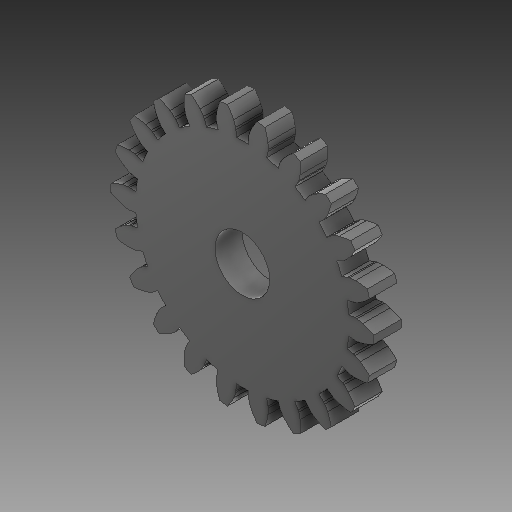
# Autodesk Inventor part: 歯車m2.z22
Saved by Autodesk Inventor 2020 (Build 240168000, 168)
## iProperties
Created: 2019-09-03
Part Number: 歯車m2.z22
Material: アセタール樹脂、黒
Document SubType Name: Modeling
Designer: 雪村
Density: 1.425 g/cm^3
Appearance: 滑らか - 黒
Mass: 6.34973 g
Surface Area: 52.6764 cm^2
Volume: 4.45595 cm^3
Description: ジュラコン 5t
Author: 雪村
Autodesk Inventor part; units mm, degrees
ref_plane "YZ Plane" through (0, 0, 0) normal (1, 0, 0) x (0, 1, 0)
ref_plane "XZ Plane" through (0, 0, 0) normal (0, 1, 0) x (-1, 0, 0)
ref_plane "XY Plane" through (0, 0, 0) normal (0, 0, 1) x (1, 0, 0)
sketch "スケッチ1" plane through (0, 0, 0) normal (0, 0, 1) x (1, 0, 0)
  arc A0 (1.2256, 20.9678) -> (1.1673, 20.6403) centre (3.2398, 20.4403) ccw
  arc A1 (1.5912, 21.9922) -> (1.2256, 20.9678) centre (6.7837, 19.5615) ccw
  arc A2 (2.7153, 23.8459) -> (1.5912, 21.9922) centre (10.6032, 17.7949) ccw
  arc A3 (-4.7313, 20.4638) -> (-4.695, 20.1331) centre (-2.6501, 20.5251) ccw
  arc A4 (-4.6691, 21.5497) -> (-4.7313, 20.4638) centre (0.9978, 20.6803) ccw
  arc A5 (-4.1128, 23.645) -> (-4.6691, 21.5497) centre (5.1603, 20.0614) ccw
  arc A6 (-10.305, 18.3019) -> (-10.1769, 17.9948) centre (-8.3254, 18.9471) ccw
  arc A7 (-10.5512, 19.3613) -> (-10.305, 18.3019) centre (-4.8689, 20.1238) ccw
  arc A8 (-10.6078, 21.5285) -> (-10.5512, 19.3613) centre (-0.7007, 20.7026) ccw
  arc A9 (-15.0438, 14.6573) -> (-14.8344, 14.3987) centre (-13.3261, 15.834) ccw
  arc A10 (-15.5785, 15.6044) -> (-15.0438, 14.6573) centre (-10.3412, 17.9369) ccw
  arc A11 (-16.2434, 17.6679) -> (-15.5785, 15.6044) centre (-6.5049, 19.6666) ccw
  arc A12 (-18.5639, 9.8252) -> (-18.2901, 9.6361) centre (-17.2473, 11.4383) ccw
  arc A13 (-19.3438, 10.5833) -> (-18.5639, 9.8252) centre (-14.9757, 14.2969) ccw
  arc A14 (-20.563, 12.3759) -> (-19.3438, 10.5833) centre (-11.7821, 17.0373) ccw
  arc A15 (-20.58, 4.1972) -> (-20.264, 4.0929) centre (-19.7712, 6.1158) ccw
  arc A16 (-21.5419, 4.7049) -> (-20.58, 4.1972) centre (-18.397, 9.4986) ccw
  arc A17 (-23.2167, 6.0813) -> (-21.5419, 4.7049) centre (-16.1048, 13.0278) ccw
  arc A18 (-20.9288, -1.7709) -> (-20.5963, -1.782) centre (-20.6933, 0.2979) ccw
  arc A19 (-21.9948, -1.5548) -> (-20.9288, -1.7709) centre (-20.3278, 3.9308) ccw
  arc A20 (-23.9896, -0.7059) -> (-21.9948, -1.5548) centre (-19.1228, 7.9628) ccw
  arc A21 (-19.5822, -7.5955) -> (-19.26, -7.5124) centre (-19.939, -5.5442) ccw
  arc A22 (-20.6658, -7.6884) -> (-19.5822, -7.5955) centre (-20.6119, -1.9555) ccw
  arc A23 (-22.819, -7.436) -> (-20.6658, -7.6884) centre (-20.5916, 2.2527) ccw
  arc A24 (-16.649, -12.8047) -> (-16.3633, -12.6343) centre (-17.5694, -10.9371) ccw
  arc A25 (-17.6626, -13.1992) -> (-16.649, -12.8047) centre (-19.226, -7.6833) ccw
  arc A26 (-19.7997, -13.5636) -> (-17.6626, -13.1992) centre (-20.3921, -3.6398) ccw
  arc A27 (-12.3671, -16.9766) -> (-12.141, -16.7326) centre (-13.7764, -15.4439) ccw
  arc A28 (-13.2285, -17.6407) -> (-12.3671, -16.9766) centre (-16.2826, -12.7886) ccw
  arc A29 (-15.1764, -18.5924) -> (-13.2285, -17.6407) centre (-18.5406, -9.2375) ccw
  arc A30 (-7.0833, -19.7732) -> (-6.9351, -19.4753) centre (-8.8673, -18.6996) ccw
  arc A31 (-7.7227, -20.653) -> (-7.0833, -19.7732) centre (-12.0201, -16.858) ccw
  arc A32 (-9.3235, -22.115) -> (-7.7227, -20.653) centre (-15.1871, -14.0868) ccw
  arc A33 (-1.2256, -20.9678) -> (-1.1673, -20.6403) centre (-3.2398, -20.4403) ccw
  arc A34 (-1.5912, -21.9922) -> (-1.2256, -20.9678) centre (-6.7837, -19.5615) ccw
  arc A35 (-2.7153, -23.8459) -> (-1.5912, -21.9922) centre (-10.6032, -17.7949) ccw
  arc A36 (4.7313, -20.4638) -> (4.695, -20.1331) centre (2.6501, -20.5251) ccw
  arc A37 (4.6691, -21.5497) -> (4.7313, -20.4638) centre (-0.9978, -20.6803) ccw
  arc A38 (4.1128, -23.645) -> (4.6691, -21.5497) centre (-5.1603, -20.0614) ccw
  arc A39 (10.305, -18.3019) -> (10.1769, -17.9948) centre (8.3254, -18.9471) ccw
  arc A40 (10.5512, -19.3613) -> (10.305, -18.3019) centre (4.8689, -20.1238) ccw
  arc A41 (10.6078, -21.5285) -> (10.5512, -19.3613) centre (0.7007, -20.7026) ccw
  arc A42 (15.0438, -14.6573) -> (14.8344, -14.3987) centre (13.3261, -15.834) ccw
  arc A43 (15.5785, -15.6044) -> (15.0438, -14.6573) centre (10.3412, -17.9369) ccw
  arc A44 (16.2434, -17.6679) -> (15.5785, -15.6044) centre (6.5049, -19.6666) ccw
  arc A45 (18.5639, -9.8252) -> (18.2901, -9.6361) centre (17.2473, -11.4383) ccw
  arc A46 (19.3438, -10.5833) -> (18.5639, -9.8252) centre (14.9757, -14.2969) ccw
  arc A47 (20.563, -12.3759) -> (19.3438, -10.5833) centre (11.7821, -17.0373) ccw
  arc A48 (20.58, -4.1972) -> (20.264, -4.0929) centre (19.7712, -6.1158) ccw
  arc A49 (21.5419, -4.7049) -> (20.58, -4.1972) centre (18.397, -9.4986) ccw
  arc A50 (23.2167, -6.0813) -> (21.5419, -4.7049) centre (16.1048, -13.0278) ccw
  arc A51 (20.9288, 1.7709) -> (20.5963, 1.782) centre (20.6933, -0.2979) ccw
  arc A52 (21.9948, 1.5548) -> (20.9288, 1.7709) centre (20.3278, -3.9308) ccw
  arc A53 (23.9896, 0.7059) -> (21.9948, 1.5548) centre (19.1228, -7.9628) ccw
  arc A54 (19.5822, 7.5955) -> (19.26, 7.5124) centre (19.939, 5.5442) ccw
  arc A55 (20.6658, 7.6884) -> (19.5822, 7.5955) centre (20.6119, 1.9555) ccw
  arc A56 (22.819, 7.436) -> (20.6658, 7.6884) centre (20.5916, -2.2527) ccw
  arc A57 (16.649, 12.8047) -> (16.3633, 12.6343) centre (17.5694, 10.9371) ccw
  arc A58 (17.6626, 13.1992) -> (16.649, 12.8047) centre (19.226, 7.6833) ccw
  arc A59 (19.7997, 13.5636) -> (17.6626, 13.1992) centre (20.3921, 3.6398) ccw
  arc A60 (12.3671, 16.9766) -> (12.141, 16.7326) centre (13.7764, 15.4439) ccw
  arc A61 (13.2285, 17.6407) -> (12.3671, 16.9766) centre (16.2826, 12.7886) ccw
  arc A62 (15.1764, 18.5924) -> (13.2285, 17.6407) centre (18.5406, 9.2375) ccw
  arc A63 (7.0833, 19.7732) -> (6.9351, 19.4753) centre (8.8673, 18.6996) ccw
  arc A64 (7.7227, 20.653) -> (7.0833, 19.7732) centre (12.0201, 16.858) ccw
  arc A65 (9.3235, 22.115) -> (7.7227, 20.653) centre (15.1871, 14.0868) ccw
  arc A66 (-1.1673, 20.6403) -> (-1.2256, 20.9678) centre (-3.2398, 20.4403) ccw
  arc A67 (-1.2256, 20.9678) -> (-1.5912, 21.9922) centre (-6.7837, 19.5615) ccw
  arc A68 (-1.5912, 21.9922) -> (-2.7153, 23.8459) centre (-10.6032, 17.7949) ccw
  arc A69 (-6.9351, 19.4753) -> (-7.0833, 19.7732) centre (-8.8673, 18.6996) ccw
  arc A70 (-7.0833, 19.7732) -> (-7.7227, 20.653) centre (-12.0201, 16.858) ccw
  arc A71 (-7.7227, 20.653) -> (-9.3235, 22.115) centre (-15.1871, 14.0868) ccw
  arc A72 (-12.141, 16.7326) -> (-12.3671, 16.9766) centre (-13.7764, 15.4439) ccw
  arc A73 (-12.3671, 16.9766) -> (-13.2285, 17.6407) centre (-16.2826, 12.7886) ccw
  arc A74 (-13.2285, 17.6407) -> (-15.1764, 18.5924) centre (-18.5406, 9.2375) ccw
  arc A75 (-16.3633, 12.6343) -> (-16.649, 12.8047) centre (-17.5694, 10.9371) ccw
  arc A76 (-16.649, 12.8047) -> (-17.6626, 13.1992) centre (-19.226, 7.6833) ccw
  arc A77 (-17.6626, 13.1992) -> (-19.7997, 13.5636) centre (-20.3921, 3.6398) ccw
  arc A78 (-19.26, 7.5124) -> (-19.5822, 7.5955) centre (-19.939, 5.5442) ccw
  arc A79 (-19.5822, 7.5955) -> (-20.6658, 7.6884) centre (-20.6119, 1.9555) ccw
  arc A80 (-20.6658, 7.6884) -> (-22.819, 7.436) centre (-20.5916, -2.2527) ccw
  arc A81 (-20.5963, 1.782) -> (-20.9288, 1.7709) centre (-20.6933, -0.2979) ccw
  arc A82 (-20.9288, 1.7709) -> (-21.9948, 1.5548) centre (-20.3278, -3.9308) ccw
  arc A83 (-21.9948, 1.5548) -> (-23.9896, 0.7059) centre (-19.1228, -7.9628) ccw
  arc A84 (-20.264, -4.0929) -> (-20.58, -4.1972) centre (-19.7712, -6.1158) ccw
  arc A85 (-20.58, -4.1972) -> (-21.5419, -4.7049) centre (-18.397, -9.4986) ccw
  arc A86 (-21.5419, -4.7049) -> (-23.2167, -6.0813) centre (-16.1048, -13.0278) ccw
  arc A87 (-18.2901, -9.6361) -> (-18.5639, -9.8252) centre (-17.2473, -11.4383) ccw
  arc A88 (-18.5639, -9.8252) -> (-19.3438, -10.5833) centre (-14.9757, -14.2969) ccw
  arc A89 (-19.3438, -10.5833) -> (-20.563, -12.3759) centre (-11.7821, -17.0373) ccw
  arc A90 (-14.8344, -14.3987) -> (-15.0438, -14.6573) centre (-13.3261, -15.834) ccw
  arc A91 (-15.0438, -14.6573) -> (-15.5785, -15.6044) centre (-10.3412, -17.9369) ccw
  arc A92 (-15.5785, -15.6044) -> (-16.2434, -17.6679) centre (-6.5049, -19.6666) ccw
  arc A93 (-10.1769, -17.9948) -> (-10.305, -18.3019) centre (-8.3254, -18.9471) ccw
  arc A94 (-10.305, -18.3019) -> (-10.5512, -19.3613) centre (-4.8689, -20.1238) ccw
  arc A95 (-10.5512, -19.3613) -> (-10.6078, -21.5285) centre (-0.7007, -20.7026) ccw
  arc A96 (-4.695, -20.1331) -> (-4.7313, -20.4638) centre (-2.6501, -20.5251) ccw
  arc A97 (-4.7313, -20.4638) -> (-4.6691, -21.5497) centre (0.9978, -20.6803) ccw
  arc A98 (-4.6691, -21.5497) -> (-4.1128, -23.645) centre (5.1603, -20.0614) ccw
  arc A99 (1.1673, -20.6403) -> (1.2256, -20.9678) centre (3.2398, -20.4403) ccw
  arc A100 (1.2256, -20.9678) -> (1.5912, -21.9922) centre (6.7837, -19.5615) ccw
  arc A101 (1.5912, -21.9922) -> (2.7153, -23.8459) centre (10.6032, -17.7949) ccw
  arc A102 (6.9351, -19.4753) -> (7.0833, -19.7732) centre (8.8673, -18.6996) ccw
  arc A103 (7.0833, -19.7732) -> (7.7227, -20.653) centre (12.0201, -16.858) ccw
  arc A104 (7.7227, -20.653) -> (9.3235, -22.115) centre (15.1871, -14.0868) ccw
  arc A105 (12.141, -16.7326) -> (12.3671, -16.9766) centre (13.7764, -15.4439) ccw
  arc A106 (12.3671, -16.9766) -> (13.2285, -17.6407) centre (16.2826, -12.7886) ccw
  arc A107 (13.2285, -17.6407) -> (15.1764, -18.5924) centre (18.5406, -9.2375) ccw
  arc A108 (16.3633, -12.6343) -> (16.649, -12.8047) centre (17.5694, -10.9371) ccw
  arc A109 (16.649, -12.8047) -> (17.6626, -13.1992) centre (19.226, -7.6833) ccw
  arc A110 (17.6626, -13.1992) -> (19.7997, -13.5636) centre (20.3921, -3.6398) ccw
  arc A111 (19.26, -7.5124) -> (19.5822, -7.5955) centre (19.939, -5.5442) ccw
  arc A112 (19.5822, -7.5955) -> (20.6658, -7.6884) centre (20.6119, -1.9555) ccw
  arc A113 (20.6658, -7.6884) -> (22.819, -7.436) centre (20.5916, 2.2527) ccw
  arc A114 (20.5963, -1.782) -> (20.9288, -1.7709) centre (20.6933, 0.2979) ccw
  arc A115 (20.9288, -1.7709) -> (21.9948, -1.5548) centre (20.3278, 3.9308) ccw
  arc A116 (21.9948, -1.5548) -> (23.9896, -0.7059) centre (19.1228, 7.9628) ccw
  arc A117 (20.264, 4.0929) -> (20.58, 4.1972) centre (19.7712, 6.1158) ccw
  arc A118 (20.58, 4.1972) -> (21.5419, 4.7049) centre (18.397, 9.4986) ccw
  arc A119 (21.5419, 4.7049) -> (23.2167, 6.0813) centre (16.1048, 13.0278) ccw
  arc A120 (18.2901, 9.6361) -> (18.5639, 9.8252) centre (17.2473, 11.4383) ccw
  arc A121 (18.5639, 9.8252) -> (19.3438, 10.5833) centre (14.9757, 14.2969) ccw
  arc A122 (19.3438, 10.5833) -> (20.563, 12.3759) centre (11.7821, 17.0373) ccw
  arc A123 (14.8344, 14.3987) -> (15.0438, 14.6573) centre (13.3261, 15.834) ccw
  arc A124 (15.0438, 14.6573) -> (15.5785, 15.6044) centre (10.3412, 17.9369) ccw
  arc A125 (15.5785, 15.6044) -> (16.2434, 17.6679) centre (6.5049, 19.6666) ccw
  arc A126 (10.1769, 17.9948) -> (10.305, 18.3019) centre (8.3254, 18.9471) ccw
  arc A127 (10.305, 18.3019) -> (10.5512, 19.3613) centre (4.8689, 20.1238) ccw
  arc A128 (10.5512, 19.3613) -> (10.6078, 21.5285) centre (0.7007, 20.7026) ccw
  arc A129 (4.695, 20.1331) -> (4.7313, 20.4638) centre (2.6501, 20.5251) ccw
  arc A130 (4.7313, 20.4638) -> (4.6691, 21.5497) centre (-0.9978, 20.6803) ccw
  arc A131 (4.6691, 21.5497) -> (4.1128, 23.645) centre (-5.1603, 20.0614) ccw
  arc A132 (1.1011, 19.4689) -> (-1.1011, 19.4689) centre (0, 0) ccw
  arc A133 (-4.4285, 18.9905) -> (-6.5415, 18.3701) centre (0, 0) ccw
  arc A134 (-9.5994, 16.9736) -> (-11.452, 15.783) centre (0, 0) ccw
  arc A135 (-13.9926, 13.5815) -> (-15.4347, 11.9173) centre (0, 0) ccw
  arc A136 (-17.2521, 9.0892) -> (-18.1669, 7.0861) centre (0, 0) ccw
  arc A137 (-19.114, 3.8606) -> (-19.4274, 1.6808) centre (0, 0) ccw
  arc A138 (-19.4274, -1.6808) -> (-19.114, -3.8606) centre (0, 0) ccw
  arc A139 (-18.1669, -7.0861) -> (-17.2521, -9.0892) centre (0, 0) ccw
  arc A140 (-15.4347, -11.9173) -> (-13.9926, -13.5815) centre (0, 0) ccw
  arc A141 (-11.452, -15.783) -> (-9.5994, -16.9736) centre (0, 0) ccw
  arc A142 (-6.5415, -18.3701) -> (-4.4285, -18.9905) centre (0, 0) ccw
  arc A143 (-1.1011, -19.4689) -> (1.1011, -19.4689) centre (0, 0) ccw
  arc A144 (4.4285, -18.9905) -> (6.5415, -18.3701) centre (0, 0) ccw
  arc A145 (9.5994, -16.9736) -> (11.452, -15.783) centre (0, 0) ccw
  arc A146 (13.9926, -13.5815) -> (15.4347, -11.9173) centre (0, 0) ccw
  arc A147 (17.2521, -9.0892) -> (18.1669, -7.0861) centre (0, 0) ccw
  arc A148 (19.114, -3.8606) -> (19.4274, -1.6808) centre (0, 0) ccw
  arc A149 (19.4274, 1.6808) -> (19.114, 3.8606) centre (0, 0) ccw
  arc A150 (18.1669, 7.0861) -> (17.2521, 9.0892) centre (0, 0) ccw
  arc A151 (15.4347, 11.9173) -> (13.9926, 13.5815) centre (0, 0) ccw
  arc A152 (11.452, 15.783) -> (9.5994, 16.9736) centre (0, 0) ccw
  arc A153 (6.5415, 18.3701) -> (4.4285, 18.9905) centre (0, 0) ccw
  arc A154 (-2.7153, 23.8459) -> (-4.1128, 23.645) centre (0, 0) ccw
  arc A155 (-9.3235, 22.115) -> (-10.6078, 21.5285) centre (0, 0) ccw
  arc A156 (-15.1764, 18.5924) -> (-16.2434, 17.6679) centre (0, 0) ccw
  arc A157 (-19.7997, 13.5636) -> (-20.563, 12.3759) centre (0, 0) ccw
  arc A158 (-22.819, 7.436) -> (-23.2167, 6.0813) centre (0, 0) ccw
  arc A159 (-23.9896, 0.7059) -> (-23.9896, -0.7059) centre (0, 0) ccw
  arc A160 (-23.2167, -6.0813) -> (-22.819, -7.436) centre (0, 0) ccw
  arc A161 (-20.563, -12.3759) -> (-19.7997, -13.5636) centre (0, 0) ccw
  arc A162 (-16.2434, -17.6679) -> (-15.1764, -18.5924) centre (0, 0) ccw
  arc A163 (-10.6078, -21.5285) -> (-9.3235, -22.115) centre (0, 0) ccw
  arc A164 (-4.1128, -23.645) -> (-2.7153, -23.8459) centre (0, 0) ccw
  arc A165 (2.7153, -23.8459) -> (4.1128, -23.645) centre (0, 0) ccw
  arc A166 (9.3235, -22.115) -> (10.6078, -21.5285) centre (0, 0) ccw
  arc A167 (15.1764, -18.5924) -> (16.2434, -17.6679) centre (0, 0) ccw
  arc A168 (19.7997, -13.5636) -> (20.563, -12.3759) centre (0, 0) ccw
  arc A169 (22.819, -7.436) -> (23.2167, -6.0813) centre (0, 0) ccw
  arc A170 (23.9896, -0.7059) -> (23.9896, 0.7059) centre (0, 0) ccw
  arc A171 (23.2167, 6.0813) -> (22.819, 7.436) centre (0, 0) ccw
  arc A172 (20.563, 12.3759) -> (19.7997, 13.5636) centre (0, 0) ccw
  arc A173 (16.2434, 17.6679) -> (15.1764, 18.5924) centre (0, 0) ccw
  arc A174 (10.6078, 21.5285) -> (9.3235, 22.115) centre (0, 0) ccw
  arc A175 (4.1128, 23.645) -> (2.7153, 23.8459) centre (0, 0) ccw
  line L0 (1.1011, 19.4689) -> (1.1673, 20.6403)
  line L1 (-4.4285, 18.9905) -> (-4.695, 20.1331)
  line L2 (-9.5994, 16.9736) -> (-10.1769, 17.9948)
  line L3 (-13.9926, 13.5815) -> (-14.8344, 14.3987)
  line L4 (-17.2521, 9.0892) -> (-18.2901, 9.6361)
  line L5 (-19.114, 3.8606) -> (-20.264, 4.0929)
  line L6 (-19.4274, -1.6808) -> (-20.5963, -1.782)
  line L7 (-18.1669, -7.0861) -> (-19.26, -7.5124)
  line L8 (-15.4347, -11.9173) -> (-16.3633, -12.6343)
  line L9 (-11.452, -15.783) -> (-12.141, -16.7326)
  line L10 (-6.5415, -18.3701) -> (-6.9351, -19.4753)
  line L11 (-1.1011, -19.4689) -> (-1.1673, -20.6403)
  line L12 (4.4285, -18.9905) -> (4.695, -20.1331)
  line L13 (9.5994, -16.9736) -> (10.1769, -17.9948)
  line L14 (13.9926, -13.5815) -> (14.8344, -14.3987)
  line L15 (17.2521, -9.0892) -> (18.2901, -9.6361)
  line L16 (19.114, -3.8606) -> (20.264, -4.0929)
  line L17 (19.4274, 1.6808) -> (20.5963, 1.782)
  line L18 (18.1669, 7.0861) -> (19.26, 7.5124)
  line L19 (15.4347, 11.9173) -> (16.3633, 12.6343)
  line L20 (11.452, 15.783) -> (12.141, 16.7326)
  line L21 (6.5415, 18.3701) -> (6.9351, 19.4753)
  line L22 (-1.1011, 19.4689) -> (-1.1673, 20.6403)
  line L23 (-6.5415, 18.3701) -> (-6.9351, 19.4753)
  line L24 (-11.452, 15.783) -> (-12.141, 16.7326)
  line L25 (-15.4347, 11.9173) -> (-16.3633, 12.6343)
  line L26 (-18.1669, 7.0861) -> (-19.26, 7.5124)
  line L27 (-19.4274, 1.6808) -> (-20.5963, 1.782)
  line L28 (-19.114, -3.8606) -> (-20.264, -4.0929)
  line L29 (-17.2521, -9.0892) -> (-18.2901, -9.6361)
  line L30 (-13.9926, -13.5815) -> (-14.8344, -14.3987)
  line L31 (-9.5994, -16.9736) -> (-10.1769, -17.9948)
  line L32 (-4.4285, -18.9905) -> (-4.695, -20.1331)
  line L33 (1.1011, -19.4689) -> (1.1673, -20.6403)
  line L34 (6.5415, -18.3701) -> (6.9351, -19.4753)
  line L35 (11.452, -15.783) -> (12.141, -16.7326)
  line L36 (15.4347, -11.9173) -> (16.3633, -12.6343)
  line L37 (18.1669, -7.0861) -> (19.26, -7.5124)
  line L38 (19.4274, -1.6808) -> (20.5963, -1.782)
  line L39 (19.114, 3.8606) -> (20.264, 4.0929)
  line L40 (17.2521, 9.0892) -> (18.2901, 9.6361)
  line L41 (13.9926, 13.5815) -> (14.8344, 14.3987)
  line L42 (9.5994, 16.9736) -> (10.1769, 17.9948)
  line L43 (4.4285, 18.9905) -> (4.695, 20.1331)
  line L44 (-26, 0) -> (26, 0)
  line L45 (0, -26) -> (0, 26)
  line L46 (44, 24) -> (114, 24)
  line L47 (44, 16) -> (114, 16)
  line L48 (44, 8) -> (114, 8)
  line L49 (44, 0) -> (114, 0)
  line L50 (44, -8) -> (114, -8)
  line L51 (44, -16) -> (114, -16)
  line L52 (44, -24) -> (114, -24)
  line L53 (44, -32) -> (114, -32)
  line L54 (44, -40) -> (114, -40)
  line L55 (44, -48) -> (114, -48)
  line L56 (44, -56) -> (114, -56)
  line L57 (44, -64) -> (114, -64)
  line L58 (44, -72) -> (114, -72)
  line L59 (44, 24) -> (44, -72)
  line L60 (114, 24) -> (114, -72)
  line L61 (79, 16) -> (79, -72)
  point P0 (0, 0)
  point P1 (50, 18)
  point P2 (52.5, 10)
  point P3 (52.5, 2)
  point P4 (50, -6)
  point P5 (52.5, -14)
  point P6 (47.5, -22)
  point P7 (50, -30)
  point P8 (50, -38)
  point P9 (50, -46)
  point P10 (52.5, -54)
  point P11 (52.5, -62)
  point P12 (50, -70)
  point P13 (80, 10)
  point P14 (95, 2)
  point P15 (96.25, -6)
  point P16 (92.5, -14)
  point P17 (95, -22)
  point P18 (88.75, -30)
  point P19 (95, -38)
  point P20 (95, -46)
  point P21 (90, -54)
  point P22 (1, 39.5)
  point P23 (1, 33.5)
  point P24 (17.1875, 39.5)
  point P25 (19.3125, 33.5)
  constraints: 264 point on circle, 132 centre point, 120 end point, 14 horizontal, 2 horizontal alignment, 2 midpoint, 2 vertical, 2 vertical alignment, 767 other
extrude "押し出し1" add sketch "スケッチ1" along normal blind 5 contours A1 A2 A175 A131 A130 A129 L43 A153 L21 A63 A64 A65 A174 A128 A127 A126 L42 A152 L20 A60 A61 A62 A173 A125 A124 A123 L41 A151 L19 A57 A58 A59 A172 A122 A121 A120 L40 A150 L18 A54 A55 A56 A171 A119 A118 A117 L39 A149 L17 A51 A52 A53 A170 L44 L45 A132 L0 A0 | L45 L44 A159 A83 A82 A81 L27 A137 L5 A15 A16 A17 A158 A80 A79 A78 L26 A136 L4 A12 A13 A14 A157 A77 A76 A75 L25 A135 L3 A9 A10 A11 A156 A74 A73 A72 L24 A134 L2 A6 A7 A8 A155 A71 A70 A69 L23 A133 L1 A3 A4 A5 A154 A68 A67 A66 L22 A132 | L45 A143 L11 A33 A34 A35 A164 A98 A97 A96 L32 A142 L10 A30 A31 A32 A163 A95 A94 A93 L31 A141 L9 A27 A28 A29 A162 A92 A91 A90 L30 A140 L8 A24 A25 A26 A161 A89 A88 A87 L29 A139 L7 A21 A22 A23 A160 A86 A85 A84 L28 A138 L6 A18 A19 A20 A159 L44 | L44 A170 A116 A115 A114 L38 A148 L16 A48 A49 A50 A169 A113 A112 A111 L37 A147 L15 A45 A46 A47 A168 A110 A109 A108 L36 A146 L14 A42 A43 A44 A167 A107 A106 A105 L35 A145 L13 A39 A40 A41 A166 A104 A103 A102 L34 A144 L12 A36 A37 A38 A165 A101 A100 A99 L33 A143 L45
sketch "スケッチ2" plane through (0, 0, 5) normal (0, 0, 1) x (1, 0, 0)
  circle A0 centre (0, 0) radius 5
  dimension "d2" = 10
  constraints: 1 centre point, 1 coincident
  measures "d2" diameter of A0
extrude "押し出し2" cut sketch "スケッチ2" against normal through all
sketch "スケッチ3" plane through (0, 0, 5) normal (0, 0, 1) x (1, 0, 0)
  circle A0 centre (0, 0) radius 8
  circle A1 centre (0, 0) radius 5
  circle A2 centre (0, 0) radius 17
  line L0 (0, 15.6403) -> (0, -15.6403)
  line L1 (-15.4429, 0) -> (15.4429, 0)
  line L2 (-1, 16.9706) -> (-1.5, 7.8581)
  line L3 (1, 16.9706) -> (1.5, 7.8581)
  line L4 (7.8581, 1.5) -> (16.9706, 1)
  line L5 (7.8581, -1.5) -> (16.9706, -1)
  circle A3 centre (0, 0) radius 8
  line L6 (1.5, -7.8581) -> (1, -16.9706)
  line L7 (-16.9706, 1) -> (-7.8581, 1.5)
  line L8 (-16.9706, -1) -> (-7.8581, -1.5)
  line L9 (-1.5, -7.8581) -> (-1, -16.9706)
  circle A4 centre (0, 0) radius 5 projected
  circle A5 centre (0, 0) radius 19.5
  point P0 (16.9761, 62.7038)
  point P1 (20.9761, 62.7038)
  point P2 (11.2302, 68.4498)
  point P3 (11.2302, 72.4498)
  point P4 (16.9761, 62.7038)
  point P5 (20.9761, 62.7038)
  point P6 (11.2302, 68.4498)
  point P7 (11.2302, 72.4498)
  point P8 (-6.5415, 18.3701)
  point P9 (-1.5, -7.8581)
  point P10 (1.5, -7.8581)
  point P11 (-7.8581, -1.5)
  point P12 (-7.8581, 1.5)
  dimension "d40" = 2.5
  dimension "d24" = 1
  dimension "d25" = 1
  dimension "d26" = 1
  dimension "d27" = 1
  dimension "d28" = 1
  dimension "d29" = 1
  dimension "d30" = 1
  dimension "d31" = 1
  dimension "d32" = 1.5
  dimension "d33" = 1.5
  dimension "d34" = 1.5
  dimension "d35" = 1.5
  dimension "d36" = 1.5
  dimension "d37" = 1.5
  dimension "d38" = 1.5
  dimension "d39" = 1.5
  dimension "d41" = 3
  constraints: 20 end point, 4 point on circle, 3 concentric, 2 centre point, 2 coincident, 2 midpoint, 1 horizontal, 1 vertical, 22 other
  measures "d24" distance from line of L0 L2.start
  measures "d25" distance from line of L3.start L0
  measures "d26" distance from line of L1 L4.end
  measures "d27" distance from line of L5.end L1
  measures "d28" distance from line of L0 L6.end
  measures "d29" distance from line of L0 L9.end
  measures "d30" distance from line of L1 L8.start
  measures "d31" distance from line of L1 L7.start
  measures "d32" distance from line of L0 L2.end
  measures "d33" distance from line of L0 L3.end
  measures "d34" distance from line of L1 L4.start
  measures "d35" distance from line of L5.start L1
  measures "d36" distance from line of L0 L6.start
  measures "d37" distance from line of L9.start L0
  measures "d38" distance from line of L1 L8.end
  measures "d39" distance from line of L1 L7.end
  measures "d41" radial gap between concentric circles of A0 A1
extrude "押し出し3" cut sketch "スケッチ3" against normal through all contours A0 L3 A2 L4 | L5 A2 L6 A0 | A0 L7 A2 L2 | L9 A2 L8 A0
fillet "フィレット1" radius 2 16 edges at (-16.9706, 1, 2.5) (-16.9706, -1, 2.5) (-7.8581, -1.5, 2.5) (-7.8581, 1.5, 2.5) (-1.5, 7.8581, 2.5) (1.5, 7.8581, 2.5) (16.9706, 1, 2.5) (16.9706, -1, 2.5) (7.8581, -1.5, 2.5) (7.8581, 1.5, 2.5) (1.5, -7.8581, 2.5) (-1.5, -7.8581, 2.5) (-1, -16.9706, 2.5) (1, -16.9706, 2.5) (-1, 16.9706, 2.5) (1, 16.9706, 2.5)
sketch "スケッチ4" plane through (0, 0, 5) normal (0, 0, 1) x (1, 0, 0)
  line L0 (9.288, -1.4215) -> (14.5604, -1.1322) projected
  arc A0 (16.626, -3.5465) -> (14.5604, -1.1322) centre (14.67, -3.1292) ccw projected
  arc A1 (3.5465, -16.626) -> (16.626, -3.5465) centre (0, 0) ccw projected
  arc A2 (1.1322, -14.5604) -> (3.5465, -16.626) centre (3.1292, -14.67) ccw projected
  line L1 (1.1322, -14.5604) -> (1.4215, -9.288) projected
  arc A3 (2.7348, -7.518) -> (1.4215, -9.288) centre (3.4185, -9.3975) ccw projected
  arc A4 (2.7348, -7.518) -> (7.518, -2.7348) centre (0, 0) ccw projected
  arc A5 (9.288, -1.4215) -> (7.518, -2.7348) centre (9.3975, -3.4185) ccw projected
  arc A6 (16.626, 3.5465) -> (3.5465, 16.626) centre (0, 0) ccw projected
  arc A7 (14.5604, 1.1322) -> (16.626, 3.5465) centre (14.67, 3.1292) ccw projected
  line L2 (14.5604, 1.1322) -> (9.288, 1.4215) projected
  arc A8 (7.518, 2.7348) -> (9.288, 1.4215) centre (9.3975, 3.4185) ccw projected
  arc A9 (7.518, 2.7348) -> (2.7348, 7.518) centre (0, 0) ccw projected
  arc A10 (1.4215, 9.288) -> (2.7348, 7.518) centre (3.4185, 9.3975) ccw projected
  line L3 (1.4215, 9.288) -> (1.1322, 14.5604) projected
  arc A11 (3.5465, 16.626) -> (1.1322, 14.5604) centre (3.1292, 14.67) ccw projected
  arc A12 (-7.518, -2.7348) -> (-2.7348, -7.518) centre (0, 0) ccw projected
  arc A13 (-1.4215, -9.288) -> (-2.7348, -7.518) centre (-3.4185, -9.3975) ccw projected
  line L4 (-1.4215, -9.288) -> (-1.1322, -14.5604) projected
  arc A14 (-3.5465, -16.626) -> (-1.1322, -14.5604) centre (-3.1292, -14.67) ccw projected
  arc A15 (-16.626, -3.5465) -> (-3.5465, -16.626) centre (0, 0) ccw projected
  arc A16 (-14.5604, -1.1322) -> (-16.626, -3.5465) centre (-14.67, -3.1292) ccw projected
  line L5 (-14.5604, -1.1322) -> (-9.288, -1.4215) projected
  arc A17 (-7.518, -2.7348) -> (-9.288, -1.4215) centre (-9.3975, -3.4185) ccw projected
  line L6 (-1.1322, 14.5604) -> (-1.4215, 9.288) projected
  arc A18 (-2.7348, 7.518) -> (-1.4215, 9.288) centre (-3.4185, 9.3975) ccw projected
  arc A19 (-2.7348, 7.518) -> (-7.518, 2.7348) centre (0, 0) ccw projected
  arc A20 (-9.288, 1.4215) -> (-7.518, 2.7348) centre (-9.3975, 3.4185) ccw projected
  line L7 (-9.288, 1.4215) -> (-14.5604, 1.1322) projected
  arc A21 (-16.626, 3.5465) -> (-14.5604, 1.1322) centre (-14.67, 3.1292) ccw projected
  arc A22 (-3.5465, 16.626) -> (-16.626, 3.5465) centre (0, 0) ccw projected
  arc A23 (-1.1322, 14.5604) -> (-3.5465, 16.626) centre (-3.1292, 14.67) ccw projected
  circle A24 centre (0, 0) radius 5 projected
  arc A25 (-9.3235, 22.115) -> (-10.6078, 21.5285) centre (0, 0) ccw projected
  arc A26 (-10.6078, 21.5285) -> (-10.5512, 19.3613) centre (-0.7007, 20.7026) ccw projected
  arc A27 (-10.5512, 19.3613) -> (-10.305, 18.3019) centre (-4.8689, 20.1238) ccw projected
  arc A28 (-10.305, 18.3019) -> (-10.1769, 17.9948) centre (-8.3254, 18.9471) ccw projected
  line L8 (-10.1769, 17.9948) -> (-9.5994, 16.9736) projected
  arc A29 (-9.5994, 16.9736) -> (-11.452, 15.783) centre (0, 0) ccw projected
  line L9 (-11.452, 15.783) -> (-12.141, 16.7326) projected
  arc A30 (-12.141, 16.7326) -> (-12.3671, 16.9766) centre (-13.7764, 15.4439) ccw projected
  arc A31 (-12.3671, 16.9766) -> (-13.2285, 17.6407) centre (-16.2826, 12.7886) ccw projected
  arc A32 (-13.2285, 17.6407) -> (-15.1764, 18.5924) centre (-18.5406, 9.2375) ccw projected
  arc A33 (-15.1764, 18.5924) -> (-16.2434, 17.6679) centre (0, 0) ccw projected
  arc A34 (-16.2434, 17.6679) -> (-15.5785, 15.6044) centre (-6.5049, 19.6666) ccw projected
  arc A35 (-15.5785, 15.6044) -> (-15.0438, 14.6573) centre (-10.3412, 17.9369) ccw projected
  arc A36 (-15.0438, 14.6573) -> (-14.8344, 14.3987) centre (-13.3261, 15.834) ccw projected
  line L10 (-14.8344, 14.3987) -> (-13.9926, 13.5815) projected
  arc A37 (-13.9926, 13.5815) -> (-15.4347, 11.9173) centre (0, 0) ccw projected
  line L11 (-15.4347, 11.9173) -> (-16.3633, 12.6343) projected
  arc A38 (-16.3633, 12.6343) -> (-16.649, 12.8047) centre (-17.5694, 10.9371) ccw projected
  arc A39 (-16.649, 12.8047) -> (-17.6626, 13.1992) centre (-19.226, 7.6833) ccw projected
  arc A40 (-17.6626, 13.1992) -> (-19.7997, 13.5636) centre (-20.3921, 3.6398) ccw projected
  arc A41 (-19.7997, 13.5636) -> (-20.563, 12.3759) centre (0, 0) ccw projected
  arc A42 (-20.563, 12.3759) -> (-19.3438, 10.5833) centre (-11.7821, 17.0373) ccw projected
  arc A43 (-19.3438, 10.5833) -> (-18.5639, 9.8252) centre (-14.9757, 14.2969) ccw projected
  arc A44 (-18.5639, 9.8252) -> (-18.2901, 9.6361) centre (-17.2473, 11.4383) ccw projected
  line L12 (-18.2901, 9.6361) -> (-17.2521, 9.0892) projected
  arc A45 (-17.2521, 9.0892) -> (-18.1669, 7.0861) centre (0, 0) ccw projected
  line L13 (-18.1669, 7.0861) -> (-19.26, 7.5124) projected
  arc A46 (-19.26, 7.5124) -> (-19.5822, 7.5955) centre (-19.939, 5.5442) ccw projected
  arc A47 (-19.5822, 7.5955) -> (-20.6658, 7.6884) centre (-20.6119, 1.9555) ccw projected
  arc A48 (-20.6658, 7.6884) -> (-22.819, 7.436) centre (-20.5916, -2.2527) ccw projected
  arc A49 (-22.819, 7.436) -> (-23.2167, 6.0813) centre (0, 0) ccw projected
  arc A50 (-23.2167, 6.0813) -> (-21.5419, 4.7049) centre (-16.1048, 13.0278) ccw projected
  arc A51 (-21.5419, 4.7049) -> (-20.58, 4.1972) centre (-18.397, 9.4986) ccw projected
  arc A52 (-20.58, 4.1972) -> (-20.264, 4.0929) centre (-19.7712, 6.1158) ccw projected
  line L14 (-20.264, 4.0929) -> (-19.114, 3.8606) projected
  arc A53 (-19.114, 3.8606) -> (-19.4274, 1.6808) centre (0, 0) ccw projected
  line L15 (-19.4274, 1.6808) -> (-20.5963, 1.782) projected
  arc A54 (-20.5963, 1.782) -> (-20.9288, 1.7709) centre (-20.6933, -0.2979) ccw projected
  arc A55 (-20.9288, 1.7709) -> (-21.9948, 1.5548) centre (-20.3278, -3.9308) ccw projected
  arc A56 (-21.9948, 1.5548) -> (-23.9896, 0.7059) centre (-19.1228, -7.9628) ccw projected
  arc A57 (-23.9896, 0.7059) -> (-23.9896, -0.7059) centre (0, 0) ccw projected
  arc A58 (-23.9896, -0.7059) -> (-21.9948, -1.5548) centre (-19.1228, 7.9628) ccw projected
  arc A59 (-21.9948, -1.5548) -> (-20.9288, -1.7709) centre (-20.3278, 3.9308) ccw projected
  arc A60 (-20.9288, -1.7709) -> (-20.5963, -1.782) centre (-20.6933, 0.2979) ccw projected
  line L16 (-20.5963, -1.782) -> (-19.4274, -1.6808) projected
  arc A61 (-19.4274, -1.6808) -> (-19.114, -3.8606) centre (0, 0) ccw projected
  line L17 (-19.114, -3.8606) -> (-20.264, -4.0929) projected
  arc A62 (-20.264, -4.0929) -> (-20.58, -4.1972) centre (-19.7712, -6.1158) ccw projected
  arc A63 (-20.58, -4.1972) -> (-21.5419, -4.7049) centre (-18.397, -9.4986) ccw projected
  arc A64 (-21.5419, -4.7049) -> (-23.2167, -6.0813) centre (-16.1048, -13.0278) ccw projected
  arc A65 (-23.2167, -6.0813) -> (-22.819, -7.436) centre (0, 0) ccw projected
  arc A66 (-22.819, -7.436) -> (-20.6658, -7.6884) centre (-20.5916, 2.2527) ccw projected
  arc A67 (-20.6658, -7.6884) -> (-19.5822, -7.5955) centre (-20.6119, -1.9555) ccw projected
  arc A68 (-19.5822, -7.5955) -> (-19.26, -7.5124) centre (-19.939, -5.5442) ccw projected
  line L18 (-19.26, -7.5124) -> (-18.1669, -7.0861) projected
  arc A69 (-18.1669, -7.0861) -> (-17.2521, -9.0892) centre (0, 0) ccw projected
  line L19 (-17.2521, -9.0892) -> (-18.2901, -9.6361) projected
  arc A70 (-18.2901, -9.6361) -> (-18.5639, -9.8252) centre (-17.2473, -11.4383) ccw projected
  arc A71 (-18.5639, -9.8252) -> (-19.3438, -10.5833) centre (-14.9757, -14.2969) ccw projected
  arc A72 (-19.3438, -10.5833) -> (-20.563, -12.3759) centre (-11.7821, -17.0373) ccw projected
  arc A73 (-20.563, -12.3759) -> (-19.7997, -13.5636) centre (0, 0) ccw projected
  arc A74 (-19.7997, -13.5636) -> (-17.6626, -13.1992) centre (-20.3921, -3.6398) ccw projected
  arc A75 (-17.6626, -13.1992) -> (-16.649, -12.8047) centre (-19.226, -7.6833) ccw projected
  arc A76 (-16.649, -12.8047) -> (-16.3633, -12.6343) centre (-17.5694, -10.9371) ccw projected
  line L20 (-16.3633, -12.6343) -> (-15.4347, -11.9173) projected
  arc A77 (-15.4347, -11.9173) -> (-13.9926, -13.5815) centre (0, 0) ccw projected
  line L21 (-13.9926, -13.5815) -> (-14.8344, -14.3987) projected
  arc A78 (-14.8344, -14.3987) -> (-15.0438, -14.6573) centre (-13.3261, -15.834) ccw projected
  arc A79 (-15.0438, -14.6573) -> (-15.5785, -15.6044) centre (-10.3412, -17.9369) ccw projected
  arc A80 (-15.5785, -15.6044) -> (-16.2434, -17.6679) centre (-6.5049, -19.6666) ccw projected
  arc A81 (-16.2434, -17.6679) -> (-15.1764, -18.5924) centre (0, 0) ccw projected
  arc A82 (-15.1764, -18.5924) -> (-13.2285, -17.6407) centre (-18.5406, -9.2375) ccw projected
  arc A83 (-13.2285, -17.6407) -> (-12.3671, -16.9766) centre (-16.2826, -12.7886) ccw projected
  arc A84 (-12.3671, -16.9766) -> (-12.141, -16.7326) centre (-13.7764, -15.4439) ccw projected
  line L22 (-12.141, -16.7326) -> (-11.452, -15.783) projected
  arc A85 (-11.452, -15.783) -> (-9.5994, -16.9736) centre (0, 0) ccw projected
  line L23 (-9.5994, -16.9736) -> (-10.1769, -17.9948) projected
  arc A86 (-10.1769, -17.9948) -> (-10.305, -18.3019) centre (-8.3254, -18.9471) ccw projected
  arc A87 (-10.305, -18.3019) -> (-10.5512, -19.3613) centre (-4.8689, -20.1238) ccw projected
  arc A88 (-10.5512, -19.3613) -> (-10.6078, -21.5285) centre (-0.7007, -20.7026) ccw projected
  arc A89 (-10.6078, -21.5285) -> (-9.3235, -22.115) centre (0, 0) ccw projected
  arc A90 (-9.3235, -22.115) -> (-7.7227, -20.653) centre (-15.1871, -14.0868) ccw projected
  arc A91 (-7.7227, -20.653) -> (-7.0833, -19.7732) centre (-12.0201, -16.858) ccw projected
  arc A92 (-7.0833, -19.7732) -> (-6.9351, -19.4753) centre (-8.8673, -18.6996) ccw projected
  line L24 (-6.9351, -19.4753) -> (-6.5415, -18.3701) projected
  arc A93 (-6.5415, -18.3701) -> (-4.4285, -18.9905) centre (0, 0) ccw projected
  line L25 (-4.4285, -18.9905) -> (-4.695, -20.1331) projected
  arc A94 (-4.695, -20.1331) -> (-4.7313, -20.4638) centre (-2.6501, -20.5251) ccw projected
  arc A95 (-4.7313, -20.4638) -> (-4.6691, -21.5497) centre (0.9978, -20.6803) ccw projected
  arc A96 (-4.6691, -21.5497) -> (-4.1128, -23.645) centre (5.1603, -20.0614) ccw projected
  arc A97 (-4.1128, -23.645) -> (-2.7153, -23.8459) centre (0, 0) ccw projected
  arc A98 (-2.7153, -23.8459) -> (-1.5912, -21.9922) centre (-10.6032, -17.7949) ccw projected
  arc A99 (-1.5912, -21.9922) -> (-1.2256, -20.9678) centre (-6.7837, -19.5615) ccw projected
  arc A100 (-1.2256, -20.9678) -> (-1.1673, -20.6403) centre (-3.2398, -20.4403) ccw projected
  line L26 (-1.1673, -20.6403) -> (-1.1011, -19.4689) projected
  arc A101 (-1.1011, -19.4689) -> (1.1011, -19.4689) centre (0, 0) ccw projected
  line L27 (1.1011, -19.4689) -> (1.1673, -20.6403) projected
  arc A102 (1.1673, -20.6403) -> (1.2256, -20.9678) centre (3.2398, -20.4403) ccw projected
  arc A103 (1.2256, -20.9678) -> (1.5912, -21.9922) centre (6.7837, -19.5615) ccw projected
  arc A104 (1.5912, -21.9922) -> (2.7153, -23.8459) centre (10.6032, -17.7949) ccw projected
  arc A105 (2.7153, -23.8459) -> (4.1128, -23.645) centre (0, 0) ccw projected
  arc A106 (4.1128, -23.645) -> (4.6691, -21.5497) centre (-5.1603, -20.0614) ccw projected
  arc A107 (4.6691, -21.5497) -> (4.7313, -20.4638) centre (-0.9978, -20.6803) ccw projected
  arc A108 (4.7313, -20.4638) -> (4.695, -20.1331) centre (2.6501, -20.5251) ccw projected
  line L28 (4.695, -20.1331) -> (4.4285, -18.9905) projected
  arc A109 (4.4285, -18.9905) -> (6.5415, -18.3701) centre (0, 0) ccw projected
  line L29 (6.5415, -18.3701) -> (6.9351, -19.4753) projected
  arc A110 (6.9351, -19.4753) -> (7.0833, -19.7732) centre (8.8673, -18.6996) ccw projected
  arc A111 (7.0833, -19.7732) -> (7.7227, -20.653) centre (12.0201, -16.858) ccw projected
  arc A112 (7.7227, -20.653) -> (9.3235, -22.115) centre (15.1871, -14.0868) ccw projected
  arc A113 (9.3235, -22.115) -> (10.6078, -21.5285) centre (0, 0) ccw projected
  arc A114 (10.6078, -21.5285) -> (10.5512, -19.3613) centre (0.7007, -20.7026) ccw projected
  arc A115 (10.5512, -19.3613) -> (10.305, -18.3019) centre (4.8689, -20.1238) ccw projected
  arc A116 (10.305, -18.3019) -> (10.1769, -17.9948) centre (8.3254, -18.9471) ccw projected
  line L30 (10.1769, -17.9948) -> (9.5994, -16.9736) projected
  arc A117 (9.5994, -16.9736) -> (11.452, -15.783) centre (0, 0) ccw projected
  line L31 (11.452, -15.783) -> (12.141, -16.7326) projected
  arc A118 (12.141, -16.7326) -> (12.3671, -16.9766) centre (13.7764, -15.4439) ccw projected
  arc A119 (12.3671, -16.9766) -> (13.2285, -17.6407) centre (16.2826, -12.7886) ccw projected
  arc A120 (13.2285, -17.6407) -> (15.1764, -18.5924) centre (18.5406, -9.2375) ccw projected
  arc A121 (15.1764, -18.5924) -> (16.2434, -17.6679) centre (0, 0) ccw projected
  arc A122 (16.2434, -17.6679) -> (15.5785, -15.6044) centre (6.5049, -19.6666) ccw projected
  arc A123 (15.5785, -15.6044) -> (15.0438, -14.6573) centre (10.3412, -17.9369) ccw projected
  arc A124 (15.0438, -14.6573) -> (14.8344, -14.3987) centre (13.3261, -15.834) ccw projected
  line L32 (14.8344, -14.3987) -> (13.9926, -13.5815) projected
  arc A125 (13.9926, -13.5815) -> (15.4347, -11.9173) centre (0, 0) ccw projected
  line L33 (15.4347, -11.9173) -> (16.3633, -12.6343) projected
  arc A126 (16.3633, -12.6343) -> (16.649, -12.8047) centre (17.5694, -10.9371) ccw projected
  arc A127 (16.649, -12.8047) -> (17.6626, -13.1992) centre (19.226, -7.6833) ccw projected
  arc A128 (17.6626, -13.1992) -> (19.7997, -13.5636) centre (20.3921, -3.6398) ccw projected
  arc A129 (19.7997, -13.5636) -> (20.563, -12.3759) centre (0, 0) ccw projected
  arc A130 (20.563, -12.3759) -> (19.3438, -10.5833) centre (11.7821, -17.0373) ccw projected
  arc A131 (19.3438, -10.5833) -> (18.5639, -9.8252) centre (14.9757, -14.2969) ccw projected
  arc A132 (18.5639, -9.8252) -> (18.2901, -9.6361) centre (17.2473, -11.4383) ccw projected
  line L34 (18.2901, -9.6361) -> (17.2521, -9.0892) projected
  arc A133 (17.2521, -9.0892) -> (18.1669, -7.0861) centre (0, 0) ccw projected
  line L35 (18.1669, -7.0861) -> (19.26, -7.5124) projected
  arc A134 (19.26, -7.5124) -> (19.5822, -7.5955) centre (19.939, -5.5442) ccw projected
  arc A135 (19.5822, -7.5955) -> (20.6658, -7.6884) centre (20.6119, -1.9555) ccw projected
  arc A136 (20.6658, -7.6884) -> (22.819, -7.436) centre (20.5916, 2.2527) ccw projected
  arc A137 (22.819, -7.436) -> (23.2167, -6.0813) centre (0, 0) ccw projected
  arc A138 (23.2167, -6.0813) -> (21.5419, -4.7049) centre (16.1048, -13.0278) ccw projected
  arc A139 (21.5419, -4.7049) -> (20.58, -4.1972) centre (18.397, -9.4986) ccw projected
  arc A140 (20.58, -4.1972) -> (20.264, -4.0929) centre (19.7712, -6.1158) ccw projected
  line L36 (20.264, -4.0929) -> (19.114, -3.8606) projected
  arc A141 (19.114, -3.8606) -> (19.4274, -1.6808) centre (0, 0) ccw projected
  line L37 (19.4274, -1.6808) -> (20.5963, -1.782) projected
  arc A142 (20.5963, -1.782) -> (20.9288, -1.7709) centre (20.6933, 0.2979) ccw projected
  arc A143 (20.9288, -1.7709) -> (21.9948, -1.5548) centre (20.3278, 3.9308) ccw projected
  arc A144 (21.9948, -1.5548) -> (23.9896, -0.7059) centre (19.1228, 7.9628) ccw projected
  arc A145 (23.9896, -0.7059) -> (23.9896, 0.7059) centre (0, 0) ccw projected
  arc A146 (23.9896, 0.7059) -> (21.9948, 1.5548) centre (19.1228, -7.9628) ccw projected
  arc A147 (21.9948, 1.5548) -> (20.9288, 1.7709) centre (20.3278, -3.9308) ccw projected
  arc A148 (20.9288, 1.7709) -> (20.5963, 1.782) centre (20.6933, -0.2979) ccw projected
  line L38 (20.5963, 1.782) -> (19.4274, 1.6808) projected
  arc A149 (19.4274, 1.6808) -> (19.114, 3.8606) centre (0, 0) ccw projected
  line L39 (19.114, 3.8606) -> (20.264, 4.0929) projected
  arc A150 (20.264, 4.0929) -> (20.58, 4.1972) centre (19.7712, 6.1158) ccw projected
  arc A151 (20.58, 4.1972) -> (21.5419, 4.7049) centre (18.397, 9.4986) ccw projected
  arc A152 (21.5419, 4.7049) -> (23.2167, 6.0813) centre (16.1048, 13.0278) ccw projected
  arc A153 (23.2167, 6.0813) -> (22.819, 7.436) centre (0, 0) ccw projected
  arc A154 (22.819, 7.436) -> (20.6658, 7.6884) centre (20.5916, -2.2527) ccw projected
  arc A155 (20.6658, 7.6884) -> (19.5822, 7.5955) centre (20.6119, 1.9555) ccw projected
  arc A156 (19.5822, 7.5955) -> (19.26, 7.5124) centre (19.939, 5.5442) ccw projected
  line L40 (19.26, 7.5124) -> (18.1669, 7.0861) projected
  arc A157 (18.1669, 7.0861) -> (17.2521, 9.0892) centre (0, 0) ccw projected
  line L41 (17.2521, 9.0892) -> (18.2901, 9.6361) projected
  arc A158 (18.2901, 9.6361) -> (18.5639, 9.8252) centre (17.2473, 11.4383) ccw projected
  arc A159 (18.5639, 9.8252) -> (19.3438, 10.5833) centre (14.9757, 14.2969) ccw projected
  arc A160 (19.3438, 10.5833) -> (20.563, 12.3759) centre (11.7821, 17.0373) ccw projected
  arc A161 (20.563, 12.3759) -> (19.7997, 13.5636) centre (0, 0) ccw projected
  arc A162 (19.7997, 13.5636) -> (17.6626, 13.1992) centre (20.3921, 3.6398) ccw projected
  arc A163 (17.6626, 13.1992) -> (16.649, 12.8047) centre (19.226, 7.6833) ccw projected
  arc A164 (16.649, 12.8047) -> (16.3633, 12.6343) centre (17.5694, 10.9371) ccw projected
  line L42 (16.3633, 12.6343) -> (15.4347, 11.9173) projected
  arc A165 (15.4347, 11.9173) -> (13.9926, 13.5815) centre (0, 0) ccw projected
  line L43 (13.9926, 13.5815) -> (14.8344, 14.3987) projected
  arc A166 (14.8344, 14.3987) -> (15.0438, 14.6573) centre (13.3261, 15.834) ccw projected
  arc A167 (15.0438, 14.6573) -> (15.5785, 15.6044) centre (10.3412, 17.9369) ccw projected
  arc A168 (15.5785, 15.6044) -> (16.2434, 17.6679) centre (6.5049, 19.6666) ccw projected
  arc A169 (16.2434, 17.6679) -> (15.1764, 18.5924) centre (0, 0) ccw projected
  arc A170 (15.1764, 18.5924) -> (13.2285, 17.6407) centre (18.5406, 9.2375) ccw projected
  arc A171 (13.2285, 17.6407) -> (12.3671, 16.9766) centre (16.2826, 12.7886) ccw projected
  arc A172 (12.3671, 16.9766) -> (12.141, 16.7326) centre (13.7764, 15.4439) ccw projected
  line L44 (12.141, 16.7326) -> (11.452, 15.783) projected
  arc A173 (11.452, 15.783) -> (9.5994, 16.9736) centre (0, 0) ccw projected
  line L45 (9.5994, 16.9736) -> (10.1769, 17.9948) projected
  arc A174 (10.1769, 17.9948) -> (10.305, 18.3019) centre (8.3254, 18.9471) ccw projected
  arc A175 (10.305, 18.3019) -> (10.5512, 19.3613) centre (4.8689, 20.1238) ccw projected
  arc A176 (10.5512, 19.3613) -> (10.6078, 21.5285) centre (0.7007, 20.7026) ccw projected
  arc A177 (10.6078, 21.5285) -> (9.3235, 22.115) centre (0, 0) ccw projected
  arc A178 (9.3235, 22.115) -> (7.7227, 20.653) centre (15.1871, 14.0868) ccw projected
  arc A179 (7.7227, 20.653) -> (7.0833, 19.7732) centre (12.0201, 16.858) ccw projected
  arc A180 (7.0833, 19.7732) -> (6.9351, 19.4753) centre (8.8673, 18.6996) ccw projected
  line L46 (6.9351, 19.4753) -> (6.5415, 18.3701) projected
  arc A181 (6.5415, 18.3701) -> (4.4285, 18.9905) centre (0, 0) ccw projected
  line L47 (4.4285, 18.9905) -> (4.695, 20.1331) projected
  arc A182 (4.695, 20.1331) -> (4.7313, 20.4638) centre (2.6501, 20.5251) ccw projected
  arc A183 (4.7313, 20.4638) -> (4.6691, 21.5497) centre (-0.9978, 20.6803) ccw projected
  arc A184 (4.6691, 21.5497) -> (4.1128, 23.645) centre (-5.1603, 20.0614) ccw projected
  arc A185 (4.1128, 23.645) -> (2.7153, 23.8459) centre (0, 0) ccw projected
  arc A186 (2.7153, 23.8459) -> (1.5912, 21.9922) centre (10.6032, 17.7949) ccw projected
  arc A187 (1.5912, 21.9922) -> (1.2256, 20.9678) centre (6.7837, 19.5615) ccw projected
  arc A188 (1.2256, 20.9678) -> (1.1673, 20.6403) centre (3.2398, 20.4403) ccw projected
  line L48 (1.1673, 20.6403) -> (1.1011, 19.4689) projected
  arc A189 (1.1011, 19.4689) -> (-1.1011, 19.4689) centre (0, 0) ccw projected
  line L49 (-1.1011, 19.4689) -> (-1.1673, 20.6403) projected
  arc A190 (-1.1673, 20.6403) -> (-1.2256, 20.9678) centre (-3.2398, 20.4403) ccw projected
  arc A191 (-1.2256, 20.9678) -> (-1.5912, 21.9922) centre (-6.7837, 19.5615) ccw projected
  arc A192 (-1.5912, 21.9922) -> (-2.7153, 23.8459) centre (-10.6032, 17.7949) ccw projected
  arc A193 (-2.7153, 23.8459) -> (-4.1128, 23.645) centre (0, 0) ccw projected
  arc A194 (-4.1128, 23.645) -> (-4.6691, 21.5497) centre (5.1603, 20.0614) ccw projected
  arc A195 (-4.6691, 21.5497) -> (-4.7313, 20.4638) centre (0.9978, 20.6803) ccw projected
  arc A196 (-4.7313, 20.4638) -> (-4.695, 20.1331) centre (-2.6501, 20.5251) ccw projected
  line L50 (-4.695, 20.1331) -> (-4.4285, 18.9905) projected
  arc A197 (-4.4285, 18.9905) -> (-6.5415, 18.3701) centre (0, 0) ccw projected
  line L51 (-6.5415, 18.3701) -> (-6.9351, 19.4753) projected
  arc A198 (-6.9351, 19.4753) -> (-7.0833, 19.7732) centre (-8.8673, 18.6996) ccw projected
  arc A199 (-7.0833, 19.7732) -> (-7.7227, 20.653) centre (-12.0201, 16.858) ccw projected
  arc A200 (-7.7227, 20.653) -> (-9.3235, 22.115) centre (-15.1871, 14.0868) ccw projected
extrude "押し出し4" add sketch "スケッチ4" against normal blind 0.7 contours L0 A0 A1 A2 L1 A3 A4 A5 | A7 L2 A8 A9 A10 L3 A11 A6 | A12 A13 L4 A14 A15 A16 L5 A17 | L6 A18 A19 A20 L7 A21 A22 A23
equation "\"d25\" = d24"
equation "\"d26\" = d25"
equation "\"d27\" = d26"
equation "\"d28\" = d27"
equation "\"d29\" = d28"
equation "\"d30\" = d25"
equation "\"d31\" = d24"
equation "\"d33\" = d32"
equation "\"d34\" = d33"
equation "\"d35\" = d34"
equation "\"d36\" = d35"
equation "\"d37\" = d35"
equation "\"d38\" = d32"
equation "\"d39\" = d38"
